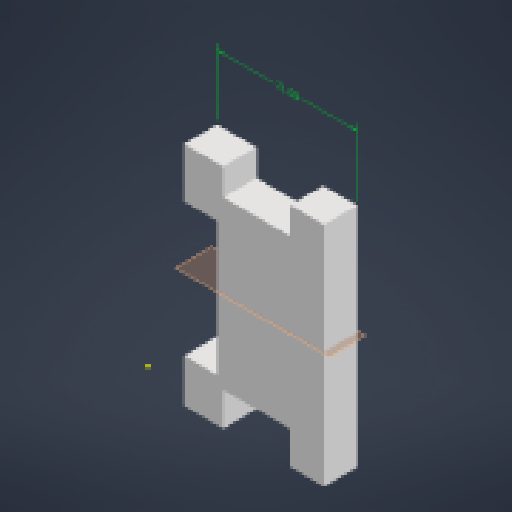
# Autodesk Inventor part: Part6
Saved by Autodesk Inventor 2026.2 (Build 302298000, 298)
## iProperties
Created: 2026-04-17
Part Number: Part6
Material: Generic
Document SubType Name: Modeling
Designer: danda
Density: 1 g/cm^3
Appearance: Default
Author: danda
Autodesk Inventor part; units mm, degrees
ref_plane "YZ Plane" through (0, 0, 0) normal (1, 0, 0) x (0, 1, 0)
ref_plane "XZ Plane" through (0, 0, 0) normal (0, 1, 0) x (-1, 0, 0)
ref_plane "XY Plane" through (0, 0, 0) normal (0, 0, 1) x (1, 0, 0)
sketch "Sketch1" plane through (0, 0, 0) normal (0, 0, 1) x (1, 0, 0)
  line L0 (5.4369, 31.5378) -> (26.4369, 31.5378)
  line L1 (26.4369, 31.5378) -> (26.4369, -2.4622)
  line L2 (26.4369, -2.4622) -> (5.4369, -2.4622)
  line L3 (5.4369, -2.4622) -> (5.4369, 31.5378)
  dimension "d3" = 21
  dimension "d4" = 34
  constraints: 8 end point, 2 parallel, 1 horizontal, 1 perpendicular
  measures "d3" distance of L1.end L2.end
  measures "d4" distance of L0.end L1.end
extrude "Extrusion1" add sketch "Sketch1" along normal blind 5
sketch "Sketch2" plane through (5.4369, -2.4622, 0) normal (0, -1, 0) x (1, 0, 0)
  line L0 (0, 5) -> (21, 5) projected
  line L1 (3, 5) -> (18.7735, 5)
  line L2 (3, 5) -> (5.8868, 0)
  line L3 (0, 0) -> (21, 0) projected
  line L4 (3, 5) -> (8.7735, 5) construction
  line L5 (18.7735, 5) -> (15.8868, 0)
  line L6 (18.7735, 5) -> (24.547, 5) construction
  line L7 (15.8868, 0) -> (5.8868, 0)
  line L8 (5.8868, 0) -> (5.8868, 5)
  line L9 (15.8868, 5) -> (15.8868, 0)
  point P0 (-5.4369, 0)
  dimension "d8" = 3
  dimension "d9" = 60
  dimension "d10" = 120
  dimension "d32" = 10
  constraints: 16 end point, 5 point on line, 2 equal length, 2 horizontal, 1 collinear, 1 midpoint, 1 perpendicular
  measures "d8" distance of L0.start L1.start
  measures "d9" angle of L2 L4
  measures "d10" angle of L5 L6
  measures "d32" distance of L5.end L2.end
extrude "Extrusion2" cut sketch "Sketch2" against normal blind 5 contours L0 L9 L3 L8
ref_plane "Work Plane1" through (5.4369, 15.0378, 0) normal (0, 1, 0) x (1, 0, 0)
mirror "Mirror1" about plane through (5.4369, 15.0378, 0) normal (0, 1, 0) of "Extrusion2"
sketch "Sketch3" plane through (5.4369, -2.4622, 0) normal (-1, 0, 0) x (0, 0, 1)
  line L0 (0, 34) -> (5, 34) projected
  line L1 (0, 1) -> (0, 34)
  line L2 (0, 34) -> (5, 34)
  line L3 (5, 34) -> (5, 0)
  line L4 (5, 6.5) -> (5, 26.5)
  line L5 (5, 6.5) -> (0, 6.5)
  line L6 (5, 6.5) -> (10, 6.5) construction
  line L7 (5, 26.5) -> (0, 26.5)
  line L8 (5, 26.5) -> (10, 26.5) construction
  line L9 (0, 26.5) -> (0, 6.5)
  dimension "d24" = 20
  dimension "d25" = 6.5
  dimension "d28" = 180
  dimension "d31" = 90
  constraints: 18 end point, 4 point on line, 2 collinear, 2 horizontal, 1 parallel, 1 vertical
  measures "d24" distance of L4.start L4.end
  measures "d25" distance of L3.end L4.start
  measures "d28" angle of L7 L8
  measures "d31" angle of L3 L5
extrude "Extrusion3" cut sketch "Sketch3" against normal blind 5 contours L7 L3 L5 L1
sketch "Sketch4" plane through (0, 0, 5) normal (0, 0, 1) x (1, 0, 0)
  point P0 (0, 0)
body "Solid1"
